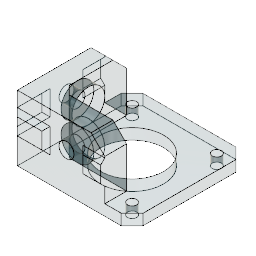
XY Motor Corner Buddy (Autodesk Fusion 360 design; units mm, degrees)
Autodesk Fusion 360 part; units mm, degrees
sketch "Sketch1" plane through (0, 0, 0) normal (0, 0, 1) x (-1, 0, 0)
  line L0 (-42, -42) -> (-42, 0)
  circle A0 centre (-36.5, -36.5) radius 1.7
  circle A1 centre (-36.5, -5.5) radius 1.7
  circle A2 centre (-5.5, -5.5) radius 1.7 construction
  circle A3 centre (-5.5, -36.5) radius 1.7
  line L1 (-5.5, -36.5) -> (-36.5, -36.5) construction
  line L2 (-36.5, -5.5) -> (-5.5, -5.5) construction
  line L3 (-36.5, -36.5) -> (-36.5, -5.5) construction
  circle A4 centre (-21, -21) radius 11.5
  line L4 (0, 0) -> (0, -42)
  line L5 (0, 0) -> (-42, 0)
  line L6 (-5.5, -5.5) -> (-36.5, -36.5) construction
  line L7 (-5.5, -36.5) -> (-5.5, -5.5) construction
  line L8 (-8, -8) -> (-32, -8)
  line L9 (-32, -8) -> (-32, 0)
  line L10 (-8, -8) -> (-8, -32)
  line L11 (-8, -32) -> (0, -32)
  line L12 (0, -42) -> (-42, -42)
  circle A5 centre (-36.5, -5.5) radius 4 construction
  circle A6 centre (-5.5, -36.5) radius 4 construction
  dimension "d1130" = 31
  dimension "d1131" = 31
  dimension "d1132" = 3.4
  dimension "d1173" = 23
  dimension "d1184" = 0
  dimension "d1185" = 0
  dimension "d1186" = 0
  dimension "d1187" = 0
  dimension "d1331" = 42
  dimension "d1332" = 42
  dimension "d1339" = 0
  dimension "d1340" = 0
  dimension "d1341" = 0
  dimension "d1342" = 0
  dimension "d1367" = 0
  dimension "d1368" = 0
  dimension "d1369" = 0
  dimension "d1370" = 0
  dimension "d1450" = 0
  dimension "d1451" = 0
  dimension "d1452" = 0
  dimension "d1453" = 0
  dimension "d1458" = 0
  dimension "d1459" = 0
  dimension "d1460" = 0
  dimension "d1461" = 0
  dimension "d1615" = 0
  dimension "d1616" = 0
  dimension "d1617" = 0
  dimension "d1618" = 0
  dimension "d2598" = 32
  dimension "d2" = 32
  dimension "d4" = 20
  dimension "d181" = 5.5
  dimension "d182" = 8
  dimension "d199" = 0
  dimension "d200" = 0
  dimension "d201" = 0
  dimension "d202" = 0
  dimension "d277" = 8
  constraint equal A0 A3
  constraint equal A2 A3
  constraint equal A1 A2
  constraint coincident A3.centre L1.start
  constraint coincident A0.centre L1.end
  constraint coincident A1.centre L2.start
  constraint coincident A2.centre L2.end
  constraint parallel L1 L2
  constraint perpendicular L1 L3
  constraint coincident L0 L5.end
  constraint perpendicular L0 L5
  constraint coincident L0.end L5.end
  constraint perpendicular L7 L8
  constraint coincident L5 L9.end
  constraint perpendicular L5 L9
  constraint vertical L7
  constraint coincident L4 L11.end
  constraint perpendicular L4 L11
  constraint equal L9 L11
  constraint equal L8 L10
  constraint perpendicular L0 L12
  constraint horizontal L5
  constraint vertical L4
  constraint coincident L4.start L5.start
  constraint symmetric L0.end L4.end L6
  constraint midpoint A4.centre L6
  constraint concentric A1 A5
  constraint concentric A3 A6
  constraint equal A5 A6
  measures "d1130" distance of A0.centre A3.centre
  measures "d1131" distance of A0.centre A1.centre
  measures "d1132" diameter of A0
  measures "d1173" diameter of A4
  measures "d1331" horizontal distance of L0.start L4.end
  measures "d1332" vertical distance of L0.start L0.end
  measures "d2598" horizontal distance of L4.start L9.end
  measures "d2" vertical distance of L4.start L11.end
  measures "d181" distance of L4 L7
  measures "d182" diameter of A5
  measures "d277" distance of L8.end L9.end
extrude "Extrude1" add sketch "Sketch1" against normal blind 4
chamfer "Chamfer6" distance 4 angle 45 3 edges at (42, 0, -2) (0, 42, -2) (42, 42, -2)
extrude "Extrude6" add sketch "Sketch1" along normal blind 20 contours L4 L5 L8 L9 L10 L11
sketch "Sketch6" plane through (32, 0, 0) normal (1, 0, 0) x (0, 1, 0)
  line L0 (0, 0) -> (8, 0)
  line L1 (8, 0) -> (8, 20)
  line L2 (8, 20) -> (0, 20)
  line L3 (0, 20) -> (0, 0)
  line L4 (0, 10) -> (-1.5, 10) construction
  line L5 (0, 14.5) -> (-1.5, 13)
  line L6 (-1.5, 13) -> (-1.5, 7)
  line L7 (-1.5, 7) -> (0, 5.5)
  dimension "d7" = 1.5
  dimension "d8" = 6
  constraint midpoint L3 L4.start
  constraint horizontal L4
  constraint coincident L3 L5.start
  constraint parallel L3 L6
  constraint coincident L3 L7.end
  constraint perpendicular L5 L7
  constraint midpoint L4.end L6
  constraint symmetric L4 L5.start L7.end
  measures "d7" distance of L4.start L4.end
  measures "d8" vertical distance of L5.end L6.end
extrude "Extrude11" add sketch "Sketch6" against normal blind 8 contours L3 L5 L6 L7
extrude "Extrude12" add 1 faces at (24, -0.5, 11) along direction (-1, 0, 0) blind 12 from surface at 12
ref_plane "WorkPlane1" through (0, 0, 8) normal (0.707107, -0.707107, 0) x (0, 0, -1)
mirror "Mirror1" about plane through (0, 0, 8) normal (0.707107, -0.707107, 0) of "Extrude11", "Extrude12"
hole "Hole3" at (18, 8, 10) direction (0, -1, 0) diameter 5.5 depth 19 tip angle 118 counterbore diameter 12 counterbore depth 4
hole "Hole4" at (8, 18, 10) direction (-1, 0, 0) diameter 5.5 depth 12 tip angle 118 counterbore diameter 12 counterbore depth 4
chamfer "Chamfer4" distance 5 angle 45 2 edges at (32, 4, 20) (4, 32, 20)
chamfer "Chamfer7" distance 1.5 angle 45 6 edges at (12, -1.5, 10) (24, -1.5, 10) (-1.5, 12, 10) (-1.5, 24, 10) (0, -1.5, 10) (-1.5, 0, 10)
chamfer "Chamfer8" distance 3 angle 45 1 edges at (8, 8, 10)
equation "d1131 = d1130"
equation "d1332 = d1331"
equation "d2 = d2598"
named bodies: "Motor Corner Buddy"
